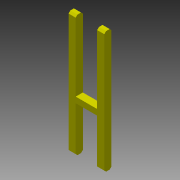
# Autodesk Inventor part: T-1S64-01-02-S
Saved by Autodesk Inventor 2014 SP2 (Build 180246200, 246)
## iProperties
Created: 2019-03-13
Part Number: T-1S64-01-02-S
Material: Generic
Catalog Web Link: www.cadenas.de
Description: T-1S64-Pins
Vendor: SAMTEC
Document SubType Name: Modeling
Designer: psadmin
Manufacturer: SAMTEC
Mass: 0.00925613 g
Surface Area: 0.594872 cm^2
Volume: 0.00925613 cm^3
Density: 1 g/cm^3
Appearance: PSOLRGB-255-255-0
Category: PARTsolutions
Company: SAMTEC
Title: T-1S64-01-02-S
Author: Cadenas PARTsolutions
Comments: Pins
PSOL_IDENT_0: {$CADENAS_DATA\23d-libs\samtec\modelling\ipl1\parts\ipl1_pins.prj},189 {VTYP=3D},{NB=T-1S64-01-02-S}
PSOL_IDENT_1: ,{LINA=T-1S64-01-02-S},{NN=T-1S64},{DATE=31.07.2018 08:10:50},{GEOMDATE=31.07.2018 07:50:48},{VERSIO
PSOL_IDENT_2: N=},{LINEID=10},{WBVAR=POS,LS,ROPT,TOPT,POPT},{WBNUMERIC=}  {NB=T-1S64-01-02-S},{LINA=T-1S64-01-02-S
PSOL_IDENT_3: },{KT=DUMMY},{PN=T-1S64-01-02-S},{SERIES=IPL1},{POSALG= '02' , '-02' ,  '03' , '-03' , '04' , '-04'
PSOL_IDENT_4: , '05' , '-05' , '06' , '-06' , '07' , '-07' , '08' , '-08'  ,  '09' , '-09' ,  '10' , '-10' ,  '11'
PSOL_IDENT_5: , '-11' , '12' , '-12'  ,  '13' , '-13' ,  '14' , '-14' , '15' , '-15' , '16' , '-16'  ,  '17' , '-
PSOL_IDENT_6: 17' ,  '18' , '-18' , '19' , '-19' ,  '20' , '-20' ,  '21' , '-21' , '22' , '-22' , '23' , '-23' , '
PSOL_IDENT_7: 24' , '-24' ,  '25' , '-25'  },{POS=02},{LS=01},{ROPTALG=   'S'  ,  '-S - Single Row'  ,   'D'  ,   '
PSOL_IDENT_8: -D - Double Row'    },{ROPT=S},{TOPTALG=  ''  , 'Not Selected'  ,   'RA'  , '-RA - Right Angle'   ,
PSOL_IDENT_9: 'RE1'  , '-RE1 - Right Angle Elevated'    },{TOPT=},{POPT=},{POPTALG=  ''  ,  'Not Available'   },
PSOL_IDENT_10: {A=0.345},{B=0.320},{E=0.230},{W=0.2400},{PINS=2},{PINL=0.120},{PINW=0.025},{PINT=0.025},{PITCH=0.10
PSOL_IDENT_11: 00},{POPTN=2},{EVEN=1},{TOPTPN=},{POPTALG2=  '' , 'Not Selected' ,  '01' , '01' , '02' , '02'   },{P
PSOL_IDENT_12: OPTPN=}
NN: T-1S64
NT: Pins
NB: T-1S64-01-02-S
NBSYN: $PN.
LINA: T-1S64-01-02-S
PN: T-1S64-01-02-S
SERIES: IPL1
POS: -02
LS: -01
ROPT: -S - Single Row
TOPT: Not Selected
POPT: Not Available
A: 0.345
B: 0.32
E: 0.23
W: 0.24
PINL: 0.12
PINW: 0.025
PINT: 0.025
PITCH: 0.1
SUPPLIER: SAMTEC
ARTICLENO: T-1S64-01-02-S
BOMINFO: T-1S64-01-02-S
CREATOR: CADENAS GmbH
Autodesk Inventor part; units mm, degrees
ref_plane "YZ Plane" through (0, 0, 0) normal (1, 0, 0) x (0, 1, 0)
ref_plane "XZ Plane" through (0, 0, 0) normal (0, 1, 0) x (-1, 0, 0)
ref_plane "XY Plane" through (0, 0, 0) normal (0, 0, 1) x (1, 0, 0)
sketch "Sketch_2" plane through (0, 0, 0) normal (1, 0, 0) x (0, 1, 0)
  line L0 (7.5883, 0.0635) -> (-2.8893, 0.0635)
  line L1 (-2.8893, 0.0635) -> (-3.048, -0.0953)
  line L2 (-3.048, -0.0953) -> (-3.048, -0.4128)
  line L3 (-3.048, -0.4128) -> (-2.8893, -0.5715)
  line L4 (-2.8893, -0.5715) -> (7.5883, -0.5715)
  line L5 (7.5883, -0.5715) -> (7.747, -0.4128)
  line L6 (7.747, -0.4128) -> (7.747, -0.0953)
  line L7 (7.747, -0.0953) -> (7.5883, 0.0635)
  constraints: 16 end point
extrude "Extrusion1" add sketch "Sketch_2" along normal mid plane 3.175
sketch "Sketch_10" plane through (0, 0, 0) normal (0, 0, 1) x (1, 0, 0)
  line L0 (-3.4925, -3.556) -> (4.1275, -3.556)
  line L1 (4.1275, -3.556) -> (4.1275, -3.048)
  line L2 (4.1275, -3.048) -> (3.4925, -3.048)
  line L3 (3.4925, -3.048) -> (3.4925, 1.016)
  line L4 (3.4925, 1.016) -> (1.5875, 1.016)
  line L5 (1.5875, 1.016) -> (1.5875, -3.048)
  line L6 (1.5875, -3.048) -> (0.9525, -3.048)
  line L7 (0.9525, -3.048) -> (0.9525, 1.016)
  line L8 (0.9525, 1.016) -> (-0.9525, 1.016)
  line L9 (-0.9525, 1.016) -> (-0.9525, -3.048)
  line L10 (-0.9525, -3.048) -> (-1.5875, -3.048)
  line L11 (-1.5875, -3.048) -> (-1.5875, 1.016)
  line L12 (-1.5875, 1.016) -> (-3.4925, 1.016)
  line L13 (-3.4925, 1.016) -> (-3.4925, -3.556)
  constraints: 28 end point
extrude "Extrusion2" cut sketch "Sketch_10" along normal mid plane 6.096
sketch "Sketch_22" plane through (0, 0, 0) normal (0, 0, 1) x (1, 0, 0)
  line L0 (-3.4925, 9.652) -> (-3.4925, 1.524)
  line L1 (-3.4925, 1.524) -> (-1.5875, 1.524)
  line L2 (-1.5875, 1.524) -> (-1.5875, 9.144)
  line L3 (-1.5875, 9.144) -> (-0.9525, 9.144)
  line L4 (-0.9525, 9.144) -> (-0.9525, 1.524)
  line L5 (-0.9525, 1.524) -> (0.9525, 1.524)
  line L6 (0.9525, 1.524) -> (0.9525, 9.144)
  line L7 (0.9525, 9.144) -> (1.5875, 9.144)
  line L8 (1.5875, 9.144) -> (1.5875, 1.524)
  line L9 (1.5875, 1.524) -> (3.4925, 1.524)
  line L10 (3.4925, 1.524) -> (3.4925, 9.144)
  line L11 (3.4925, 9.144) -> (4.1275, 9.144)
  line L12 (4.1275, 9.144) -> (4.1275, 9.652)
  line L13 (4.1275, 9.652) -> (-3.4925, 9.652)
  constraints: 28 end point
extrude "Extrusion3" cut sketch "Sketch_22" along normal mid plane 6.096
ref_plane "pins_to_header_XY" through (0, 0, 0) normal (0, 1, 0) x (1, 0, 0)
ref_plane "pins_to_header_YZ" through (0, 0, 0) normal (1, 0, 0) x (0, 0, -1)
ref_plane "pins_to_header_ZX" through (0, 0, 0) normal (0, 0, -1) x (0, 1, 0)
body "Solid1"
